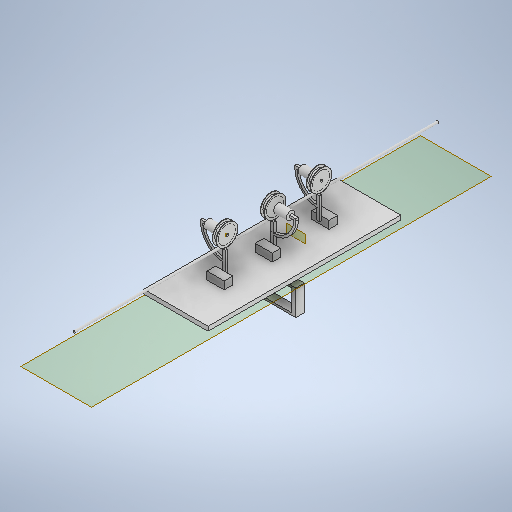
# Autodesk Inventor part: MECH
Saved by Autodesk Inventor 2025 (Build 290162000, 162)
## iProperties
Created: 2024-09-04
Part Number: MECH
Material: Generic
Document SubType Name: Modeling
Designer: sajid
Density: 1 g/cm^3
Appearance: Default
Author: sajid
Autodesk Inventor part; units mm, degrees
ref_plane "YZ Plane" through (0, 0, 0) normal (1, 0, 0) x (0, 1, 0)
ref_plane "XZ Plane" through (0, 0, 0) normal (0, 1, 0) x (-1, 0, 0)
ref_plane "XY Plane" through (0, 0, 0) normal (0, 0, 1) x (1, 0, 0)
sketch "Sketch1" plane through (0, 0, 0) normal (0, 1, 0) x (-1, 0, 0)
  line L0 (-75, 225) -> (75, 225)
  line L1 (75, 225) -> (75, -225)
  line L2 (75, -225) -> (-75, -225)
  line L3 (-75, -225) -> (-75, 225)
  line L4 (-75, 225) -> (75, -225) construction
  line L5 (75, 225) -> (-75, -225) construction
  point P0 (0, 0)
  dimension "d0" = 150
  dimension "d1" = 450
  constraints: 12 end point, 2 midpoint, 2 parallel, 1 horizontal, 1 perpendicular
  measures "d0" distance of L1.end L2.end
  measures "d1" distance of L0.end L1.end
extrude "Extrusion1" add sketch "Sketch1" along normal blind 10
sketch "Sketch2" plane through (0, 10, 0) normal (0, 1, 0) x (1, 0, 0)
  line L0 (20, -132.5) -> (-20, -132.5)
  line L1 (-20, -132.5) -> (-20, -112.5)
  line L2 (-20, -112.5) -> (20, -112.5)
  line L3 (20, -112.5) -> (20, -132.5)
  line L4 (20, 132.5) -> (-20, 132.5)
  line L5 (-20, 132.5) -> (-20, 112.5)
  line L6 (-20, 112.5) -> (20, 112.5)
  line L7 (20, 112.5) -> (20, 132.5)
  line L8 (20, -20) -> (-20, -20)
  line L9 (-20, -20) -> (-20, 0)
  line L10 (-20, 0) -> (20, 0)
  line L11 (20, 0) -> (20, -20)
  point P0 (0, 0)
  constraints: 24 end point, 4 parallel, 2 horizontal, 2 perpendicular
extrude "Extrusion2" add sketch "Sketch2" along normal blind 18
sketch "Sketch3" plane through (20, 10, 112.5) normal (0, 0, -1) x (-1, 0, 0)
  line L0 (95, 0) -> (-55, 0) projected
  line L1 (17, 61.5124) -> (17, 9)
  line L2 (17, 9) -> (23, 9)
  arc A0 (23, 35.0819) -> (75, 90) centre (20, 90) ccw
  arc A1 (23, 40.0901) -> (70, 90) centre (20, 90) ccw
  line L3 (23, 9) -> (23, 35.0819)
  line L4 (23, 40.0901) -> (23, 61.5124)
  line L5 (23, 61.5124) -> (17, 61.5124)
  line L6 (70, 90) -> (30, 90)
  line L7 (30, 90) -> (30, 95)
  line L8 (30, 95) -> (75, 95)
  line L9 (75, 95) -> (75, 90)
  point P0 (20, -10)
  point P1 (20, 35)
  constraints: 18 end point, 4 parallel, 4 perpendicular, 4 point on circle, 2 centre point, 1 coincident, 1 horizontal
extrude "Extrusion3" add sketch "Sketch3" along normal blind 5
sketch "Sketch4" plane through (-10, 100, 112.5) normal (1, 0, 0) x (0, 0, -1)
  line L0 (0, 0) -> (5, 0) projected
  line L1 (5, 5) -> (5, 0) projected
  line L2 (0, 0) -> (5, 0)
  line L3 (5, 0) -> (5, 5)
  line L4 (5, 5) -> (0, 5)
  line L5 (0, 5) -> (0, 0)
  circle A0 centre (2.5, 2.5) radius 10
  point P0 (112.5, -100)
  constraints: 8 end point, 2 parallel, 1 centre point, 1 horizontal, 1 perpendicular
extrude "Extrusion4" add sketch "Sketch4" against normal blind 30 contours L5 L4 L1 L0 | A0
sketch "Sketch5" plane through (-10, 102.5, 110) normal (1, 0, 0) x (0, 0, -1)
  circle A0 centre (0, 0) radius 2.5
  line L0 (2.5, -2.5) -> (2.5, 2.5) projected
  point P0 (110, -102.5)
  constraints: 1 centre point, 1 tangent
extrude "Extrusion5" add sketch "Sketch5" along normal blind 16
ref_plane "Work Plane1" through (-0.5, 102.5, 110) normal (1, 0, 0) x (0, 0, -1)
sketch "Sketch6" plane through (-0.5, 102.5, 110) normal (1, 0, 0) x (0, 0, -1)
  circle A0 centre (0, 0) radius 2.5 projected
  circle A1 centre (0, 0) radius 20
  point P0 (110, -102.5)
  dimension "d25" = 40
  constraints: 1 centre point, 1 coincident
  measures "d25" diameter of A1
ref_plane "Work Plane2" through (3.5, 102.5, 110) normal (1, 0, 0) x (0, 0, -1)
sketch "Sketch7" plane through (3.5, 102.5, 110) normal (1, 0, 0) x (0, 0, -1)
  circle A0 centre (0, 0) radius 25
  point P0 (110, -102.5)
  dimension "d27" = 50
  constraints: 1 centre point
  measures "d27" diameter of A0
ref_plane "Work Plane3" through (-4.5, 102.5, 110) normal (1, 0, 0) x (0, 0, -1)
sketch "Sketch8" plane through (-4.5, 102.5, 110) normal (1, 0, 0) x (0, 0, -1)
  circle A0 centre (0, 0) radius 25
  point P0 (110, -102.5)
  dimension "d29" = 50
  constraints: 1 centre point
  measures "d29" diameter of A0
extrude "Extrusion6" add sketch "Sketch7" along normal blind 1
extrude "Extrusion7" add sketch "Sketch8" against normal blind 1
extrude "Extrusion8" add sketch "Sketch6" along normal mid plane 8.5 contours A0 | A1
mirror "Mirror1" about plane through (0, 0, 0) normal (0, 0, 1) of "Extrusion3"
mirror "Mirror2" about plane through (0, 0, 0) normal (0, 0, 1) of "Extrusion4"
mirror "Mirror3" about plane through (0, 0, 0) normal (0, 0, 1) of "Extrusion8", "Extrusion7", "Extrusion6"
mirror "Mirror4" about plane through (0, 0, 0) normal (0, 0, 1) of "Extrusion5"
sketch "Sketch9" plane through (20, 10, 0) normal (0, 0, -1) x (-1, 0, 0)
  point P0 (20, -10)
sketch "Sketch10" plane through (20, 10, 0) normal (0, 0, -1) x (-1, 0, 0)
  line L0 (18.1935, 8.9026) -> (22.9808, 8.9026)
  arc A0 (22.9808, 34.9845) -> (23, 34.9855) centre (19.9808, 89.9026) ccw
  arc A1 (22.9808, 39.9927) -> (23, 39.9938) centre (19.9808, 89.9026) ccw
  line L1 (22.9808, 8.9026) -> (22.9808, 34.9845)
  line L2 (22.9808, 39.9927) -> (22.9808, 61.5124)
  line L3 (22.9808, 61.5124) -> (18.1935, 61.5124)
  line L4 (69.7302, 94.9026) -> (69.7686, 94.9026)
  line L5 (23, 61.5124) -> (17, 61.5124) projected
  line L6 (17, 61.5124) -> (20, 61.5124)
  line L7 (20, 61.5124) -> (17, 61.5124)
  line L8 (22.9808, 8.9026) -> (17, 8.9026)
  line L9 (17, 61.5124) -> (18.1935, 61.5124)
  line L10 (21.8065, 8.9026) -> (17.0192, 8.9026)
  arc A2 (-34.9808, 89.9026) -> (17.0192, 34.9845) centre (20.0192, 89.9026) ccw
  arc A3 (-29.9808, 89.9026) -> (17.0192, 39.9927) centre (20.0192, 89.9026) ccw
  line L11 (17.0192, 8.9026) -> (17.0192, 34.9845)
  line L12 (17.0192, 39.9927) -> (17.0192, 61.5124)
  line L13 (17.0192, 61.5124) -> (21.8065, 61.5124)
  line L14 (-29.9808, 89.9026) -> (10.0192, 89.9026)
  line L15 (10.0192, 89.9026) -> (10.0192, 94.9026)
  line L16 (10.0192, 94.9026) -> (-34.9808, 94.9026)
  line L17 (-34.9808, 94.9026) -> (-34.9808, 89.9026)
  line L18 (17, 61.5124) -> (23, 61.5124)
  line L19 (23, 61.5124) -> (20, 61.5124)
  line L20 (20, 61.5124) -> (23, 61.5124)
  line L21 (17.0192, 8.9026) -> (23, 8.9026)
  line L22 (23, 8.9026) -> (23, 61.5124)
  line L23 (23, 61.5124) -> (21.8065, 61.5124)
  line L24 (17, 8.9026) -> (17, 34.9855)
  line L25 (17, 39.9938) -> (17, 61.5124)
  point P0 (20, -10)
  point P1 (19.4869, -10.1944)
  point P2 (25.0913, 34.0235)
  point P3 (74.9808, 94.9026)
  point P4 (14.9087, 34.0235)
  point P5 (17.0192, 8.9026)
  constraints: 50 end point, 12 point on circle, 5 perpendicular, 4 centre point, 4 point on line, 2 coincident, 1 horizontal, 1 midpoint
sketch "Sketch11" plane through (20, 10, 0) normal (0, 0, -1) x (-1, 0, 0)
  point P0 (20, -10)
extrude "Extrusion9" add sketch "Sketch10" along normal blind 6 contours L8 L11 A2 L17 L16 L15 L14 A3 L12 L5 L3 L2 A1 L22 A0 L1 L0
sketch "Sketch12" plane through (9.9808, 99.9026, 0) normal (-1, 0, 0) x (0, 0, 1)
  circle A0 centre (-3, 2.5) radius 10
  point P0 (0, -99.9026)
  dimension "d38" = 20
  constraints: 1 centre point
  measures "d38" diameter of A0
extrude "Extrusion10" add sketch "Sketch12" against normal blind 30
ref_plane "Work Plane4" through (20, 10, -56.25) normal (0, 0, -1) x (-1, 0, 0)
mirror "Mirror5" about plane through (20, 10, -56.25) normal (0, 0, -1) of "Extrusion5", "Mirror4"
mirror "Mirror6" about plane through (20, 10, -56.25) normal (0, 0, -1) of "Extrusion8", "Extrusion7", "Extrusion6", "Mirror3"
sketch "Sketch13" plane through (6, 102.5, -222.5) normal (1, 0, 0) x (0, 0, -1)
  circle A0 centre (0, 0) radius 2.5 projected
  circle A1 centre (0, 0) radius 46.6761
  point P0 (-222.5, -102.5)
  constraints: 1 centre point, 1 coincident
extrude "Extrusion11" cut sketch "Sketch13" along normal mid plane 30 contours A0 | A1
sketch "Sketch14" plane through (-9, 102.5, -222.5) normal (1, 0, 0) x (0, 0, -1)
  circle A0 centre (0, 0) radius 4.9458
  point P0 (-222.5, -102.5)
  constraints: 1 centre point
extrude "Extrusion12" cut sketch "Sketch14" along normal mid plane 30
sketch "Sketch15" plane through (20, 10, 112.5) normal (0, 0, 1) x (1, 0, 0)
  line L0 (-24.5, 72.5) -> (-16.5, 72.5) projected
  circle A0 centre (-20.5, 70) radius 2.5
  point P0 (-20, -10)
  constraints: 1 centre point
extrude "Extrusion13" add sketch "Sketch15" along normal blind 350 and the other way blind 499
sketch "Sketch16" plane through (0, 0, 0) normal (0, -1, 0) x (1, 0, 0)
  line L0 (37.5, 125) -> (37.5, -125)
  line L1 (-37.5, -125) -> (-37.5, 125)
  arc A0 (37.5, 125) -> (-37.5, 125) centre (0, 125) ccw
  line L2 (0, 0) -> (17.5584, 0)
  arc A1 (-37.5, -125) -> (37.5, -125) centre (0, -125) ccw
  line L3 (31.5, -125) -> (31.5, 125)
  arc A2 (31.5, 125) -> (-31.5, 125) centre (0, 125) ccw
  line L4 (-31.5, 125) -> (-31.5, -125)
  arc A3 (-31.5, -125) -> (31.5, -125) centre (0, -125) ccw
  dimension "d52" = 75
  dimension "d53" = 250
  dimension "d54" = 6
  constraints: 10 end point, 8 point on circle, 4 centre point, 2 parallel, 1 horizontal, 1 symmetric about line, 1 tangent, 4 other
  measures "d52" distance of L0.end L1.start
  measures "d53" distance of L0.start L0.end
  measures "d54" distance between parallel lines of L0 L3
extrude "Extrusion14" add sketch "Sketch16" along normal blind 20
sketch "Sketch17" plane through (37.5, 0, 125) normal (1, 0, 0) x (0, 0, -1)
  line L0 (125, 0) -> (125, -20)
  line L1 (250, -20) -> (0, -20) projected
  line L2 (25, -13.5) -> (225, -13.5)
  line L3 (225, -13.5) -> (225, -6.5)
  line L4 (225, -6.5) -> (25, -6.5)
  line L5 (25, -6.5) -> (25, -13.5)
  line L6 (25, -13.5) -> (225, -6.5) construction
  line L7 (225, -13.5) -> (25, -6.5) construction
  point P0 (125, -10)
  dimension "d57" = 200
  dimension "d58" = 7
  constraints: 14 end point, 4 midpoint, 2 parallel, 1 horizontal, 1 perpendicular
  measures "d57" distance of L4.end L3.end
  measures "d58" distance of L3.end L2.end
extrude "Extrusion15" cut sketch "Sketch17" along normal mid plane 300
sketch "Sketch18" plane through (37.5, 0, 125) normal (1, 0, 0) x (0, 0, -1)
  circle A0 centre (125, -9.9179) radius 3.4179
  point P0 (125, 0)
  constraints: 1 centre point
extrude "Extrusion16" add sketch "Sketch18" along normal blind 10 and the other way blind 85
ref_plane "Work Plane6" through (31.5, -10, -100) normal (0, -1, 0) x (1, 0, 0)
sketch "Sketch19" plane through (31.5, -10, -100) normal (0, -1, 0) x (1, 0, 0)
  line L0 (-51.5, 100) -> (-11.5, 100) projected
  circle A0 centre (-11.5, 100) radius 3.5
  line L1 (-51.5, 100) -> (-51.5, 120) projected
  circle A1 centre (-51.5, 100) radius 3.5
  point P0 (-31.5, 100)
  dimension "d65" = 7
  dimension "d66" = 7
  constraints: 2 centre point, 1 coincident
  measures "d65" diameter of A0
  measures "d66" diameter of A1
extrude "Extrusion17" add sketch "Sketch19" along normal blind 15 and the other way blind 3.5
sketch "Sketch20" plane through (20, -25, 0) normal (0, -1, 0) x (1, 0, 0)
  line L0 (-85, 10) -> (45, 10)
  line L1 (45, 10) -> (45, -10)
  line L2 (45, -10) -> (-85, -10)
  line L3 (-85, -10) -> (-85, 10)
  line L4 (-85, 10) -> (45, -10) construction
  line L5 (45, 10) -> (-85, -10) construction
  point P0 (-20, 0)
  dimension "d71" = 130
  dimension "d72" = 20
  constraints: 12 end point, 2 midpoint, 2 parallel, 1 horizontal, 1 perpendicular
  measures "d71" distance of L1.end L2.end
  measures "d72" distance of L0.end L1.end
extrude "Extrusion18" add sketch "Sketch20" along normal blind 5
sketch "Sketch21" plane through (20, -30, 0) normal (0, -1, 0) x (1, 0, 0)
  line L0 (45, 10) -> (-85, 10) projected
  line L1 (-85, -10) -> (45, -10) projected
  line L2 (-85, 10) -> (-75, 10)
  line L3 (-75, 10) -> (-75, -10)
  line L4 (-75, -10) -> (-85, -10)
  line L5 (-85, -10) -> (-85, 10)
  line L6 (45, -10) -> (45, 10) projected
  line L7 (45, 10) -> (35, 10)
  line L8 (35, 10) -> (35, -10)
  line L9 (35, -10) -> (45, -10)
  line L10 (45, -10) -> (45, 10)
  point P0 (-20, 0)
  dimension "d75" = 10
  dimension "d76" = 10
  constraints: 16 end point, 4 parallel, 2 horizontal, 2 perpendicular, 2 point on line
  measures "d75" distance of L3.end L4.end
  measures "d76" distance of L9.end L8.end
extrude "Extrusion19" add sketch "Sketch21" along normal blind 50 contours L6 L1 L8 L0 | L3 L1 L5 L0
sketch "Sketch22" plane through (20, -80, 0) normal (0, -1, 0) x (1, 0, 0)
  line L0 (45, -10) -> (45, 10) projected
  line L1 (-85, 10) -> (45, 10)
  line L2 (45, 10) -> (45, -10)
  line L3 (45, -10) -> (-85, -10)
  line L4 (-85, -10) -> (-85, 10)
  line L5 (-85, 10) -> (45, -10) construction
  line L6 (45, 10) -> (-85, -10) construction
  point P0 (-20, 0)
  constraints: 12 end point, 2 midpoint, 2 parallel, 1 horizontal, 1 perpendicular
extrude "Extrusion20" add sketch "Sketch22" along normal blind 5
sketch "Sketch23" plane through (47.5, -9.9179, 0) normal (1, 0, 0) x (0, 0, -1)
  circle A0 centre (200, 0) radius 3.5
  point P0 (0, 9.9179)
  dimension "d82" = 7
  constraints: 1 centre point
  measures "d82" diameter of A0
extrude "Extrusion21" add sketch "Sketch23" along normal blind 10 and the other way blind 20
sketch "Sketch24" plane through (27.5, -9.9179, -200) normal (-1, 0, 0) x (0, 0, 1)
  line L0 (12.5, -10) -> (-12.5, -10)
  line L1 (-12.5, -10) -> (-12.5, 10)
  line L2 (-12.5, 10) -> (12.5, 10)
  line L3 (12.5, 10) -> (12.5, -10)
  line L4 (12.5, -10) -> (-12.5, 10) construction
  line L5 (-12.5, -10) -> (12.5, 10) construction
  point P0 (200, 9.9179)
  point P1 (0, 0)
  dimension "d87" = 25
  dimension "d88" = 20
  constraints: 12 end point, 2 midpoint, 2 parallel, 1 horizontal, 1 perpendicular
  measures "d87" distance of L1.end L2.end
  measures "d88" distance of L0.end L1.end
extrude "Extrusion22" add sketch "Sketch24" along normal blind 30
ref_plane "Work Plane5" through (20, 10, -56.25) normal (0, 0, -1) x (-1, 0, 0)
body "Solid1"
